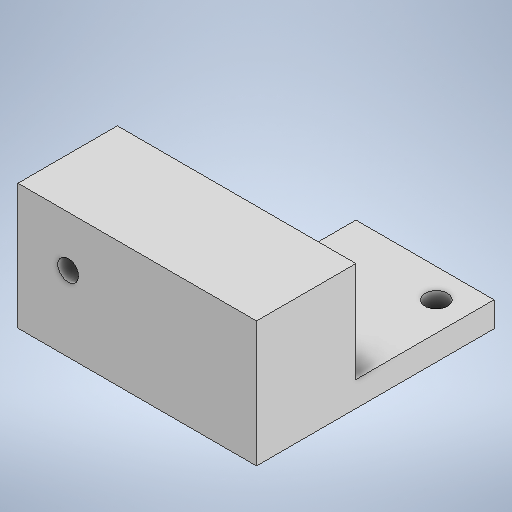
# Autodesk Inventor part: ER_Positionierungseinheit_Greifer
Saved by Autodesk Inventor 2025.1 (Build 291241000, 241)
## iProperties
Created: 2025-06-23
Part Number: ER_Positionierungseinheit_Greifer
Material: Generic
Document SubType Name: Modeling
Designer: Erik
Density: 1 g/cm^3
Appearance: Default
Author: Erik
Autodesk Inventor part; units mm, degrees
ref_plane "YZ Plane" through (0, 0, 0) normal (1, 0, 0) x (0, 1, 0)
ref_plane "XZ Plane" through (0, 0, 0) normal (0, 1, 0) x (-1, 0, 0)
ref_plane "XY Plane" through (0, 0, 0) normal (0, 0, 1) x (1, 0, 0)
sketch "Sketch1" plane through (0, 0, 0) normal (0, 1, 0) x (-1, 0, 0)
  line L0 (-13.75, 23.6455) -> (13.75, 23.6455)
  line L1 (13.75, 23.6455) -> (13.75, -23.6455)
  line L2 (13.75, -23.6455) -> (-13.75, -23.6455)
  line L3 (-13.75, -23.6455) -> (-13.75, 23.6455)
  line L4 (-13.75, 23.6455) -> (13.75, -23.6455) construction
  line L5 (13.75, 23.6455) -> (-13.75, -23.6455) construction
  point P0 (0, 0)
  dimension "d0" = 47.291
  dimension "d1" = 27.5
  constraints: 12 end point, 2 midpoint, 2 parallel, 1 horizontal, 1 perpendicular
  measures "d0" distance of L0.end L1.end
  measures "d1" distance between parallel lines of L1 L3
extrude "Extrusion1" add sketch "Sketch1" along normal blind 5
sketch "Sketch2" plane through (0, 5, 0) normal (0, 1, 0) x (1, 0, 0)
  line L0 (-13.75, 23.6455) -> (-13.75, -23.6455) projected
  line L1 (13.75, -23.6455) -> (13.75, 23.6455) projected
  line L2 (-13.75, -23.6455) -> (13.75, -23.6455)
  line L3 (13.75, -23.6455) -> (13.75, -3.8545)
  line L4 (13.75, -3.8545) -> (-13.75, -3.8545)
  line L5 (-13.75, -3.8545) -> (-13.75, -23.6455)
  point P0 (0, 0)
  dimension "d4" = 19.791
  constraints: 8 end point, 2 parallel, 1 horizontal, 1 perpendicular, 1 point on line
  measures "d4" distance between parallel lines of L4 L2
extrude "Extrusion2" add sketch "Sketch2" along normal blind 20
sketch "Sketch5" plane through (-13.75, 0, -23.6455) normal (-1, 0, 0) x (0, 0, 1)
  line L0 (47.291, 25) -> (27.5, 25) projected
  line L1 (0, 0) -> (47.291, 0) projected
  line L2 (47.291, 25) -> (27.5, 25)
  line L3 (27.5, 25) -> (27.5, 0)
  line L4 (27.5, 0) -> (47.291, 0)
  line L5 (47.291, 0) -> (47.291, 25)
  line L6 (27.5, 5) -> (27.5, 25) projected
  point P0 (23.6455, 0)
  dimension "d27" = 0
  constraints: 8 end point, 2 parallel, 1 horizontal, 1 perpendicular, 1 point on line
  measures "d27" distance between parallel lines of L6 L3
extrude "Extrusion3" add sketch "Sketch5" along normal blind 20
sketch "Sketch3" plane through (0, 0, 0) normal (0, -1, 0) x (1, 0, 0)
  line L0 (13.75, -23.6455) -> (-13.75, -23.6455) projected
  line L1 (13.75, 23.6455) -> (13.75, -23.6455) projected
  point P0 (0, 0)
  point P1 (8, -17.8955)
  point P2 (-8, -1.8955)
  dimension "d7" = 5.75
  dimension "d8" = 5.75
  dimension "d9" = 16
  dimension "d10" = 16
  measures "d7" distance from line of L0 point (8, -17.895)
  measures "d8" distance from line of L1 point (8, -17.895)
  measures "d9" horizontal distance of point (-8, -1.895) point (8, -17.895)
  measures "d10" horizontal distance of point (8, -17.895) point (-8, -1.895)
hole "Hole1" at (8, 0, -17.8955) at (-8, 0, -1.8955) direction (0, 1, 0) diameter 4.5 end through all
sketch "Sketch4" plane through (13.75, 5, 3.8545) normal (0, 0, -1) x (-1, 0, 0)
  line L0 (27.5, 0) -> (27.5, 20) projected
  line L1 (27.5, 0) -> (0, 0) projected
  line L2 (47.5, 20) -> (47.5, -5) projected
  point P0 (13.75, -5)
  point P1 (37.5, 10)
  dimension "d19" = 10
  dimension "d30" = 10
  measures "d19" distance from line of L1 point (37.5, 10)
  measures "d30" distance from line of L2 point (37.5, 10)
hole "Hole2" at (-23.75, 15, 3.8545) direction (0, 0, 1) diameter 4.134 end through all thread size "M5x0.8" class "6H" standard "ISO Metric profile"
equation "\"d8\" = d7"
body "Solid1"
